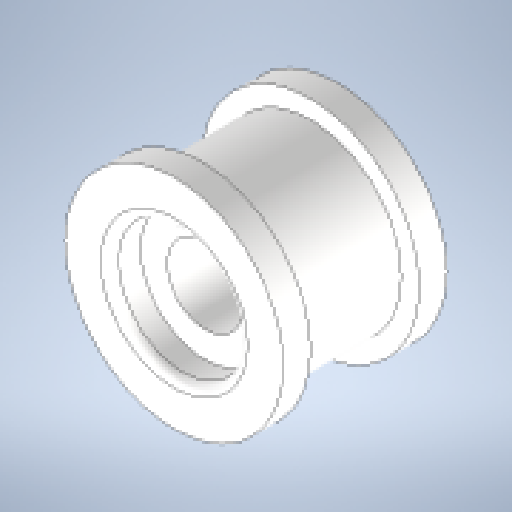
# Autodesk Inventor part: link1part5
Saved by Autodesk Inventor 2024 (Build 280153000, 153)
## iProperties
Created: 2025-02-14
Part Number: link1part5
Material: 一般
Document SubType Name: Modeling
Designer: tanoue_kota
Density: 1 g/cm^3
Appearance: 白
Mass: 5.5571 g
Surface Area: 41.2152 cm^2
Volume: 5.5571 cm^3
Author: tanoue_kota
Autodesk Inventor part; units mm, degrees
ref_plane "YZ Plane" through (0, 0, 0) normal (1, 0, 0) x (0, 1, 0)
ref_plane "XZ Plane" through (0, 0, 0) normal (0, 1, 0) x (-1, 0, 0)
ref_plane "XY Plane" through (0, 0, 0) normal (0, 0, 1) x (1, 0, 0)
sketch "スケッチ1" plane through (0, 0, 0) normal (0, 0, 1) x (1, 0, 0)
  circle A0 centre (0, 0) radius 10
  dimension "d0" = 20
  constraints: 1 centre point, 1 coincident
  measures "d0" diameter of A0
extrude "押し出し1" add sketch "スケッチ1" along normal blind 6
sketch "スケッチ2" plane through (0, 0, 0) normal (0, 0, -1) x (-1, 0, 0)
  circle A0 centre (0, 0) radius 12
  circle A1 centre (0, 0) radius 10 projected
  dimension "d17" = 2
  constraints: 1 centre point, 1 coincident
  measures "d17" radial gap between concentric circles of A1 A0
extrude "押し出し2" add sketch "スケッチ2" along normal blind 3 contours A0 | A1
sketch "スケッチ3" plane through (0, 0, -3) normal (0, 0, -1) x (-1, 0, 0)
  circle A0 centre (0, 0) radius 8
  dimension "d6" = 16
  constraints: 2 coincident, 1 centre point
  measures "d6" diameter of A0
hole "穴1" at (0, 0, -3) direction (0, 0, 1) diameter 8.4 end through all
sketch "スケッチ4" plane through (0, 0, -3) normal (0, 0, -1) x (-1, 0, 0)
  circle A0 centre (0, 0) radius 7.1
  dimension "d14" = 14.2
  constraints: 1 centre point, 1 coincident
  measures "d14" diameter of A0
extrude "押し出し3" cut sketch "スケッチ4" against normal blind 3.4
mirror "ミラー1" about plane through (0, 0, 6) normal (0, 0, 1) of "押し出し1", "押し出し2", "穴1", "押し出し3"
fillet "フィレット1" radius 1 2 edges at (7.1, 0, 15) (7.1, 0, -3)
